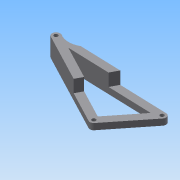
# Autodesk Inventor part: 1-1
Saved by Autodesk Inventor 2015 (Build 190159000, 159)
## iProperties
Created: 2018-05-07
Part Number: 1-1
Material: 一般
Document SubType Name: Modeling
Designer: 王博聖
Density: 1 g/cm^3
Appearance: 預設
Author: 王博聖
Autodesk Inventor part; units mm, degrees
ref_plane "YZ Plane" through (0, 0, 0) normal (1, 0, 0) x (0, 1, 0)
ref_plane "XZ Plane" through (0, 0, 0) normal (0, 1, 0) x (-1, 0, 0)
ref_plane "XY Plane" through (0, 0, 0) normal (0, 0, 1) x (1, 0, 0)
sketch "草圖1" plane through (0, 0, 0) normal (0, 0, 1) x (1, 0, 0)
  line L0 (0, 0) -> (-25.5595, 13.402) construction
  line L1 (-25.5595, 13.402) -> (9.701, 12.2296) construction
  line L2 (9.701, 12.2296) -> (0, 0) construction
  line L3 (-25.5595, 13.402) -> (0, 0) construction
  line L4 (-26.1399, 12.2949) -> (-0.5805, -1.107)
  line L5 (0.5805, 1.107) -> (-24.979, 14.509)
  arc A0 (-24.979, 14.509) -> (-26.1399, 12.2949) centre (-25.5595, 13.402) ccw
  arc A1 (-0.5805, -1.107) -> (0.5805, 1.107) centre (0, 0) ccw
  line L6 (-25.5595, 13.402) -> (9.701, 12.2296) construction
  line L7 (-25.601, 12.1527) -> (9.6595, 10.9802)
  line L8 (9.7426, 13.4789) -> (-25.5179, 14.6513)
  arc A2 (-25.5179, 14.6513) -> (-25.601, 12.1527) centre (-25.5595, 13.402) ccw
  arc A3 (9.6595, 10.9802) -> (9.7426, 13.4789) centre (9.701, 12.2296) ccw
  line L9 (9.701, 12.2296) -> (0, 0) construction
  line L10 (8.7217, 13.0064) -> (-0.9793, 0.7768)
  line L11 (0.9793, -0.7768) -> (10.6803, 11.4527)
  arc A4 (10.6803, 11.4527) -> (8.7217, 13.0064) centre (9.701, 12.2296) ccw
  arc A5 (-0.9793, 0.7768) -> (0.9793, -0.7768) centre (0, 0) ccw
  point P0 (-12.7797, 6.701)
  point P1 (-7.9292, 12.8158)
  point P2 (4.8505, 6.1148)
  dimension "d0" = 28.86
  dimension "d1" = 35.28
  dimension "d2" = 15.61
  dimension "d3" = 2.5
  dimension "d4" = 2.5
  dimension "d5" = 2.5
  constraints: 30 end point, 12 point on circle, 12 tangent, 6 centre point, 6 equal length, 3 midpoint, 1 concentric
  measures "d0" distance of L0.start L0.end
  measures "d1" distance of L0.end L1.end
  measures "d2" distance of L1.end L0.start
  measures "d3" diameter of A1
  measures "d4" diameter of A3
  measures "d5" diameter of A5
extrude "擠出1" add sketch "草圖1" along normal blind 2 contours A2 L7 L5 L10 A5 L4 | A0 L5 L7 A2 | A5 L10 L5 A1 | L8 A4 L10 L7 L5 A0 | A1 L5 L10 L7 A3 L11 | A3 L7 L10 A4
sketch "草圖2" plane through (0, 0, 2) normal (0, 0, 1) x (1, 0, 0)
  arc A0 (10.6803, 11.4527) -> (9.7426, 13.4789) centre (9.701, 12.2296) ccw projected
  arc A1 (-25.5179, 14.6513) -> (-26.1399, 12.2949) centre (-25.5595, 13.402) ccw projected
  arc A2 (-0.5805, -1.107) -> (0.9793, -0.7768) centre (0, 0) ccw projected
  circle A3 centre (0, 0) radius 0.625
  circle A4 centre (9.701, 12.2296) radius 0.625
  circle A5 centre (-25.5595, 13.402) radius 0.625
  dimension "d8" = 1.25
  dimension "d9" = 1.25
  dimension "d10" = 1.25
  constraints: 3 centre point, 3 coincident
  measures "d8" diameter of A3
  measures "d9" diameter of A4
  measures "d10" diameter of A5
extrude "擠出2" cut sketch "草圖2" against normal blind 2
sketch "草圖4" plane through (0, 0, 2) normal (0, 0, 1) x (1, 0, 0)
  circle A0 centre (-25.5595, 13.402) radius 0.625 projected
  line L0 (-0.3361, 1.5877) -> (-20.1387, 11.971) projected
  line L1 (-20.1387, 11.971) -> (7.1799, 11.0627) projected
  line L2 (9.7426, 13.4789) -> (-25.5179, 14.6513) projected
  arc A1 (-25.5179, 14.6513) -> (-26.1399, 12.2949) centre (-25.5595, 13.402) ccw projected
  line L3 (-26.1399, 12.2949) -> (-0.5805, -1.107) projected
  line L4 (-5.5082, 13.986) -> (-6.7973, 11.5274)
  line L5 (-9.4919, 6.3884) -> (-10.6529, 4.1744)
  constraints: 4 end point, 4 point on line
extrude "擠出3" add sketch "草圖4" along normal blind 4
sketch "草圖5" plane through (0, 0, 6) normal (0, 0, 1) x (1, 0, 0)
  circle A0 centre (-21.6744, 19.594) radius 6
  point P0 (0, 0)
  dimension "d17" = 12
  constraints: 1 centre point
  measures "d17" diameter of A0
extrude "擠出4" cut sketch "草圖5" against normal blind 40
sketch "草圖6" plane through (0, 0, 2) normal (0, 0, 1) x (1, 0, 0)
  arc A0 (-26.0169, 18.4563) -> (-17.0179, 18.323) centre (-21.5174, 18.3896) ccw
  line L0 (-26.0169, 18.4563) -> (-17.0179, 18.323)
  dimension "d20" = 9
  constraints: 2 end point, 2 point on circle, 1 centre point, 1 midpoint
  measures "d20" diameter of A0
sketch "草圖3" plane through (0, 0, 2) normal (0, 0, 1) x (1, 0, 0)
  line L0 (9.7426, 13.4789) -> (-25.5179, 14.6513) projected
  arc A0 (-25.5179, 14.6513) -> (-26.1399, 12.2949) centre (-25.5595, 13.402) ccw projected
  line L1 (-26.1399, 12.2949) -> (-0.5805, -1.107) projected
  line L2 (-25.5595, 17.902) -> (-25.5595, 8.902)
  arc A1 (-22.3114, 10.2875) -> (-21.1974, 14.5076) centre (-25.5595, 13.402) ccw
  arc A2 (-25.5595, 17.902) -> (-25.5595, 8.902) centre (-25.5595, 13.402) ccw
  constraints: 4 point on circle, 2 centre point, 2 end point, 2 point on line, 1 coincident, 1 vertical
